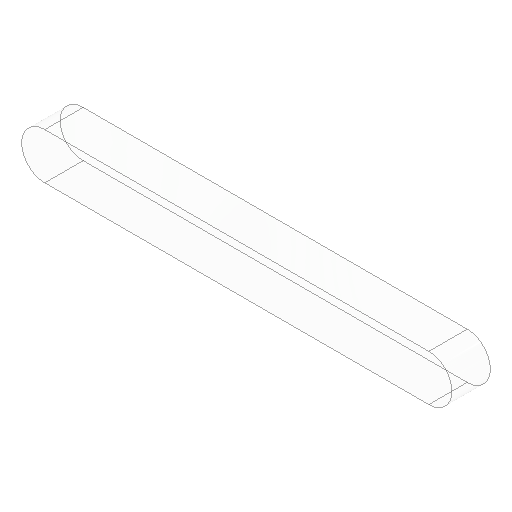
# Autodesk Inventor part: LED_Cover
Saved by Autodesk Inventor 2025.2 (Build 292293000, 293)
## iProperties
Created: 2025-03-10
Part Number: LED_Cover
Material: PMMA Plastic
Document SubType Name: Modeling
Designer: ahorat
Density: 1.188 g/cm^3
Appearance: Polycarbonate - Clear
Author: ahorat
Autodesk Inventor part; units mm, degrees
ref_plane "YZ Plane" through (0, 0, 0) normal (1, 0, 0) x (0, 1, 0)
ref_plane "XZ Plane" through (0, 0, 0) normal (0, 1, 0) x (-1, 0, 0)
ref_plane "XY Plane" through (0, 0, 0) normal (0, 0, 1) x (1, 0, 0)
sketch "Sketch1" plane through (0, 0, 0) normal (0, 0, 1) x (1, 0, 0)
  line L0 (-25, -3) -> (25, -3)
  line L1 (25, -3) -> (25, 3) construction
  line L2 (25, 3) -> (-25, 3)
  line L3 (-25, 3) -> (-25, -3) construction
  line L4 (-25, -3) -> (25, 3) construction
  line L5 (25, -3) -> (-25, 3) construction
  arc A0 (-25, 3) -> (-25, -3) centre (-25, 0) ccw
  arc A1 (25, -3) -> (25, 3) centre (25, 0) ccw
  point P0 (0, 0)
  dimension "d0" = 50
  dimension "d1" = 6
  constraints: 12 end point, 4 point on circle, 2 centre point, 2 midpoint, 2 parallel, 2 tangent, 1 horizontal, 1 perpendicular
  measures "d0" distance of L1.end L2.end
  measures "d1" distance of L0.end L1.end
extrude "Extrusion1" add sketch "Sketch1" along normal blind 5
body "Solid1"
